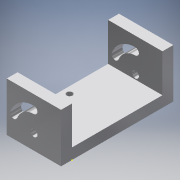
# Autodesk Inventor part: landing-gear-ublock
Saved by Autodesk Inventor 2016 (Build 200138000, 138)
## iProperties
Created: 2015-01-28
Part Number: landing-gear-ublock
Material: ABS Plastic
Document SubType Name: Modeling
Designer: Vasanth
Density: 1.06 g/cm^3
Appearance: Smooth - White
Mass: 4.80196 g
Surface Area: 33.0898 cm^2
Volume: 4.53015 cm^3
Author: Vasanth
Autodesk Inventor part; units mm, degrees
ref_plane "YZ Plane" through (0, 0, 0) normal (1, 0, 0) x (0, 1, 0)
ref_plane "XZ Plane" through (0, 0, 0) normal (0, 1, 0) x (-1, 0, 0)
ref_plane "XY Plane" through (0, 0, 0) normal (0, 0, 1) x (1, 0, 0)
sketch "Sketch1" plane through (0, 0, 0) normal (0, 1, 0) x (-1, 0, 0)
  line L0 (0, 0) -> (19.05, 0)
  line L1 (19.05, 0) -> (19.05, -31.75)
  line L2 (19.05, -31.75) -> (0, -31.75)
  line L3 (0, -31.75) -> (0, 0)
  line L4 (19.05, 0) -> (19.05, 3.81)
  line L5 (19.05, 3.81) -> (0, 3.81)
  line L6 (0, 3.81) -> (0, 0)
  line L7 (19.05, -31.75) -> (19.05, -35.56)
  line L8 (19.05, -35.56) -> (0, -35.56)
  line L9 (0, -35.56) -> (0, -31.75)
  dimension "d0" = 19.05
  dimension "d1" = 31.75
  dimension "d4" = 3.81
  dimension "d5" = 3.81
  constraints: 20 end point, 4 perpendicular, 2 parallel, 2 point on line, 1 collinear, 1 horizontal, 1 vertical
  measures "d0" distance of L1.end L2.end
  measures "d1" distance of L0.end L1.end
  measures "d4" distance of L0.end L4.end
  measures "d5" distance of L1.end L7.end
extrude "Extrusion2" add sketch "Sketch1" along normal blind 9.525
sketch "Sketch3" plane through (0, 9.525, 0) normal (0, 1, 0) x (1, 0, 0)
  line L0 (0, 0) -> (-19.05, 0)
  line L1 (-19.05, 31.75) -> (0, 31.75)
  line L2 (0, 0) -> (0, 31.75)
  line L3 (-19.05, 31.75) -> (-19.05, 0)
  point P0 (-19.05, 35.56)
  constraints: 8 end point, 1 horizontal, 1 perpendicular
extrude "Extrusion3" cut sketch "Sketch3" against normal blind 5.715
sketch "Sketch4" plane through (0, 9.525, 0) normal (0, 1, 0) x (1, 0, 0)
  line L0 (-18.8776, 0) -> (0, 0)
  line L1 (0, 0) -> (0, -3.81)
  line L2 (0, -3.81) -> (-18.8776, -3.81)
  line L3 (-19.05, 35.56) -> (0, 35.56)
  line L4 (0, 35.56) -> (0, 31.75)
  line L5 (0, 31.75) -> (-19.05, 31.75)
  line L6 (-19.05, 31.75) -> (-19.05, 35.56)
  line L7 (-18.8776, 0) -> (-19.05, 0)
  line L8 (0, 0) -> (-19.05, 0) projected
  line L9 (-19.05, 0) -> (-19.05, -3.81)
  line L10 (-18.8776, -3.81) -> (-19.05, -3.81)
  line L11 (-19.05, -3.81) -> (0, -3.81) projected
  constraints: 20 end point, 3 parallel, 3 perpendicular, 2 collinear, 2 horizontal
extrude "Extrusion4" add sketch "Sketch4" along normal blind 7.62
sketch "Sketch5" plane through (0, 3.81, 0) normal (0, 1, 0) x (1, 0, 0)
  line L0 (-19.0656, 0) -> (0, 0)
  line L1 (0, 0) -> (0, 31.75)
  line L2 (0, 31.75) -> (-19.0656, 31.75)
  line L3 (-19.0656, 31.75) -> (-19.0656, 0)
  line L4 (0, 0) -> (-19.05, 0) projected
  line L5 (-19.05, 31.75) -> (0, 31.75) projected
  line L6 (-9.525, 0) -> (22.3112, 0) construction
  line L7 (-9.525, 31.75) -> (-9.525, 0)
  line L8 (-9.525, 0) -> (-9.525, 15.875)
  line L9 (-9.525, 15.875) -> (-9.525, 31.75)
  circle A0 centre (-16.6804, 15.875) radius 1.016
  point P0 (-18.8776, 0)
  dimension "d43" = 2.032
  constraints: 16 end point, 3 midpoint, 2 horizontal, 2 parallel, 1 centre point, 1 collinear, 1 perpendicular
  measures "d43" diameter of A0
extrude "Extrusion5" cut sketch "Sketch5" against normal blind 3.81 contours A0
sketch "Sketch7" plane through (0, 0, -35.56) normal (0, 0, -1) x (-1, 0, 0)
  line L0 (19.05, 3.81) -> (0, 3.81)
  line L1 (0, 3.81) -> (0, 17.145)
  line L2 (0, 17.145) -> (19.05, 17.145)
  line L3 (19.05, 17.145) -> (19.05, 3.81)
  line L4 (19.05, 17.145) -> (0, 17.145) projected
  line L5 (19.05, 3.81) -> (0, 3.81) projected
  line L6 (0, 17.145) -> (0, 3.81) projected
  circle A0 centre (9.525, 12.3825) radius 1.016
  point P0 (0, 0)
  dimension "d42" = 2.032
  constraints: 8 end point, 2 parallel, 1 centre point, 1 horizontal, 1 perpendicular
  measures "d42" diameter of A0
extrude "Extrusion7" cut sketch "Sketch7" against normal blind 39.37 contours A0
sketch "Sketch13" plane through (-19.05, 0, 3.81) normal (0, 0, 1) x (1, 0, 0)
  arc A0 (9.5897, 13.6509) -> (9.4386, 13.6496) centre (9.525, 12.3825) ccw
  arc A1 (9.5359, 11.1125) -> (3.682, 6.9762) centre (9.5897, 4.826) ccw
  arc A2 (9.5897, 13.6509) -> (1.297, 7.8443) centre (9.5897, 4.826) ccw
  line L0 (9.5897, 4.826) -> (18.4145, 4.826) construction
  line L1 (9.5897, 4.826) -> (18.4145, 4.826) construction
  arc A3 (1.297, 7.8443) -> (3.682, 6.9762) centre (2.4895, 7.4102) ccw
  line L2 (9.5897, 4.826) -> (11.1137, 4.826) construction
  line L3 (9.5897, 6.5604) -> (9.5897, 5.3539)
  circle A4 centre (9.5897, 5.3539) radius 1.2065
  arc A5 (9.5359, 11.1125) -> (9.4386, 13.6496) centre (9.525, 12.3825) ccw
  point P0 (19.05, 0)
  point P1 (9.5897, 3.81)
  constraints: 12 point on circle, 8 end point, 6 coincident, 5 centre point, 3 horizontal, 1 tangent, 1 vertical alignment, 2 other
extrude "Extrusion14" cut sketch "Sketch13" against normal blind 76.2
sketch "Sketch21" plane through (0, 0, 0) normal (0, -1, 0) x (1, 0, 0)
  point P0 (0, 0)
body "Solid2"
